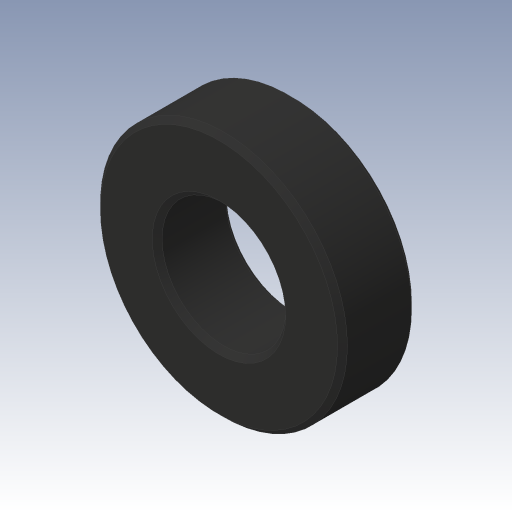
# Autodesk Inventor part: BT012_huenin20_23
Saved by Autodesk Inventor 2023.3 (Build 273359000, 359)
## iProperties
Company: HTBLA Kaindorf
RuleStatus: InUse
Created: 2023-12-01
Part Number: BT012_huenin20_23
Project: Fiberprinter-Hotend
Material: Gummi
Description: Faservorschubrad
Document SubType Name: Modeling
Designer: huenin20
Density: 0.93 g/cm^3
Appearance: Gummi - Schwarz
Mass: 0.162592 g
Surface Area: 2.4814 cm^2
Volume: 0.17483 cm^3
AfterDocNew0: iProperties-Editor_aufrufen
Author: nicob
Keywords: 2023
Autodesk Inventor part; units mm, degrees
ref_plane "YZ Plane" through (0, 0, 0) normal (1, 0, 0) x (0, 1, 0)
ref_plane "XZ Plane" through (0, 0, 0) normal (0, 1, 0) x (-1, 0, 0)
ref_plane "XY Plane" through (0, 0, 0) normal (0, 0, 1) x (1, 0, 0)
sketch "Skizze3" plane through (0, 0, 0) normal (1, 0, 0) x (0, 1, 0)
  circle A0 centre (0, 0) radius 2.5
  circle A1 centre (0, 0) radius 5
  dimension "d4" = 5
  dimension "d5" = 10
  constraints: 2 centre point, 2 coincident
  measures "d4" diameter of A0
  measures "d5" diameter of A1
extrude "Extrusion3" add sketch "Skizze3" along normal blind 3
chamfer "Fase1" distance 0.2 angle 45 4 edges at (3, -5, 0) (0, -5, 0) (3, -2.5, 0) (0, -2.5, 0)
